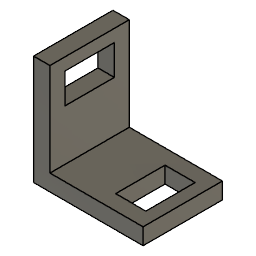
Complete printer assembly (Autodesk Fusion 360 archive; units mm, degrees)
design "T nut L clamp"
part number: 2025-12-24-15-34-34-820
Autodesk Fusion 360 part; units mm, degrees
sketch "Sketch1" plane through (0, 0, 0) normal (0, 1, 0) x (1, 0, 0)
  line L0 (0, 0) -> (3, 0)
  line L1 (3, 0) -> (3, -20)
  line L2 (3, -20) -> (0, -20)
  line L3 (0, -20) -> (0, 0)
  line L4 (0, 0) -> (20, 0)
  line L5 (20, 0) -> (20, -3)
  line L6 (20, -3) -> (0, -3)
  line L7 (0, -3) -> (0, 0)
  dimension "d1" = 20
  dimension "d2" = 3
  dimension "d3" = 20
  dimension "d4" = 3
  constraint horizontal L0
  constraint vertical L1
  constraint horizontal L2
  constraint vertical L3
  constraint coincident L0.start L3.end
  constraint horizontal L4
  constraint vertical L5
  constraint horizontal L6
  constraint vertical L7
  measures "d1" distance of L0 L2
  measures "d2" distance of L4 L6
  measures "d3" distance of L5 L7
  measures "d4" distance of L1 L3
extrude "Extrude1" add sketch "Sketch1" along normal blind 14.5
sketch "Sketch2" plane through (0, 0, 3) normal (0, 0, 1) x (-1, 0, 0)
  line L0 (-3, 0) -> (-20, 0)
  line L1 (-20, 0) -> (-20, -14.5)
  line L2 (-20, -14.5) -> (-3, -14.5)
  line L3 (-3, -14.5) -> (-3, 0)
  line L4 (-12.25, -11.75) -> (-17.75, -11.75)
  line L5 (-17.75, -11.75) -> (-17.75, -2.75)
  line L6 (-17.75, -2.75) -> (-12.25, -2.75)
  line L7 (-12.25, -2.75) -> (-12.25, -11.75)
  dimension "d7" = 5.5
  dimension "d8" = 9
  dimension "d9" = 2.75
  dimension "d10" = 2.25
  constraint horizontal L4
  constraint vertical L5
  constraint horizontal L6
  constraint vertical L7
  measures "d7" distance of L4.start L4.end
  measures "d8" distance of L4 L6
  measures "d9" distance of L0 L6
  measures "d10" distance of L1 L5
extrude "Extrude2" cut sketch "Sketch2" against normal blind 20 contours L4 L5 L6 L7
sketch "Sketch3" plane through (3, 0, 0) normal (1, 0, 0) x (0, 1, 0)
  line L0 (0, 20) -> (0, 3)
  line L1 (0, 3) -> (14.5, 3)
  line L2 (14.5, 3) -> (14.5, 20)
  line L3 (14.5, 20) -> (0, 20)
  line L4 (2.75, 17.75) -> (11.75, 17.75)
  line L5 (11.75, 17.75) -> (11.75, 12.25)
  line L6 (11.75, 12.25) -> (2.75, 12.25)
  line L7 (2.75, 12.25) -> (2.75, 17.75)
  dimension "d13" = 9
  dimension "d14" = 5.5
  dimension "d15" = 2.75
  dimension "d16" = 2.25
  constraint horizontal L4
  constraint vertical L5
  constraint horizontal L6
  constraint vertical L7
  measures "d13" distance of L4.start L4.end
  measures "d14" distance of L4 L6
  measures "d15" distance of L0 L7
  measures "d16" distance of L3 L4
extrude "Extrude3" cut sketch "Sketch3" against normal blind 20 contours L4 L5 L6 L7

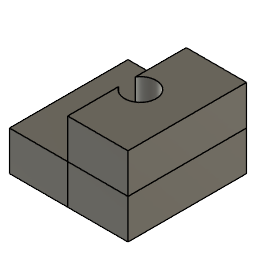
design "Z smooth rod holder"
part number: 2025-12-29-13-48-08-419
Autodesk Fusion 360 part; units mm, degrees
sketch "Sketch1" plane through (0, 0, 0) normal (0, 0, 1) x (1, 0, 0)
  line L0 (0, 0) -> (30, 0)
  line L1 (30, 0) -> (30, 30)
  line L2 (30, 30) -> (0, 30)
  line L3 (0, 30) -> (0, 0)
  circle A0 centre (13, 15) radius 2.75
  circle A1 centre (18.14, 15) radius 4
  line L4 (14.7492, 17.122) -> (14.7492, 12.878)
  line L5 (14.7492, 12.878) -> (14.7492, 0)
  line L6 (14.7492, 0) -> (14.7492, 30)
  dimension "d1" = 30
  dimension "d2" = 30
  dimension "d3" = 5.5
  dimension "d4" = 13
  dimension "d5" = 8
  dimension "d6" = 15
  dimension "d7" = 15
  dimension "d8" = 5.14
  constraint horizontal L0
  constraint vertical L1
  constraint horizontal L2
  constraint vertical L3
  constraint coincident L0.start L3.end
  constraint coincident A1 L4.start
  constraint coincident A0 L4.start
  constraint coincident A1 L4.end
  constraint coincident A0 L4.end
  constraint coincident L0 L5.end
  constraint perpendicular L0 L5
  constraint coincident L2 L6.end
  constraint perpendicular L2 L6
  measures "d1" distance of L1 L3
  measures "d2" distance of L0 L2
  measures "d3" diameter of A0
  measures "d4" distance of L3 A0.centre
  measures "d5" diameter of A1
  measures "d6" distance of L0 A0.centre
  measures "d7" distance of L0 A1.centre
  measures "d8" distance of A0.centre A1.centre
extrude "Extrude1" add sketch "Sketch1" along normal blind 10 contours L0 L2 L3 A0 L5 L6 | L0 L1 L2 A1 L5 L6 makes body 1
extrude "Extrude2" add sketch "Sketch1" along normal blind 20 separate body contours L0 L1 L2 A1 L5 L6 makes body 2

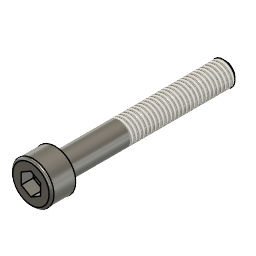
design "Hexagon Socket Head Cap Screw ISO 4762 - M5 x 35 Steel 4.6 Plain"
description: Hexagon Socket Head Cap Screw ISO 4762 - M5 x 35
part number: ISO 4762 - M5 x 35 Steel 4.6 Plain
Autodesk Fusion 360 part; units mm, degrees
sketch "Sketch1" plane through (0, 0, 0) normal (0, 1, 0) x (1, 0, 0)
  line L0 (-2.5, 0) -> (-2.5, 35)
  line L1 (-2.5, 35) -> (0, 35)
  line L2 (0, 35) -> (0, -5)
  line L3 (-2.5, 0) -> (-4.25, 0)
  line L4 (-4.25, 0) -> (-4.25, -5)
  line L5 (-4.25, -5) -> (0, -5)
  dimension "d9" = 5
  dimension "d106" = 5
  dimension "d107" = 35
  dimension "d116" = 8.5
  constraint perpendicular L0 L1
  constraint collinear origin L1.end L2.end
  constraint perpendicular L0 L3
  constraint coincident origin L3
  constraint vertical L2
  constraint coincident L2 L5.end
  constraint perpendicular L2 L5
  measures "d106" distance of L3 L5
  measures "d107" distance of origin L1
revolve "Revolve1" add sketch "Sketch1" angle 360 about axis through (0, 0, -35) along (0, 0, 1)
ref_plane "WorkPlane1" through (0, 0, 5) normal (0, 0, 1) x (1, 0, 0)
sketch "Sketch6" plane through (0, 0, 5) normal (0, 0, 1) x (1, 0, 0)
  line L0 (-2, 1.1547) -> (-2, -1.1547)
  line L1 (-2, -1.1547) -> (0, -2.3094)
  line L2 (0, -2.3094) -> (2, -1.1547)
  line L3 (2, -1.1547) -> (2, 1.1547)
  line L4 (2, 1.1547) -> (0, 2.3094)
  line L5 (0, 2.3094) -> (-2, 1.1547)
  dimension "d117" = 4
  constraint vertical L0
  measures "d117" distance of L0 L3
extrude "Extrude1" cut sketch "Sketch6" against normal blind 2.5
extrude "Extrude2" cut 1 faces at (0.6667, -0.3849, 2.5) along direction (0, 0, -1) blind 2.5 draft -85
fillet "Fillet4" radius 0.5 1 edges at (-3.9624, 1.5369, 5)
thread "Thread3" "ISO Metric profile 5.0 M5x0.8 M5x0.8 6g" major diameter 4.901 minor diameter 3.9895 pitch 0.8 angle 60 resizes the face on face at (-2.4969, 0.1246, -23.3333) from (0, 0, -13) to (0, 0, -35)
sketch "Sketch7" plane through (0, 0, 0) normal (0, 1, 0) x (1, 0, 0)
  line L0 (-2.55, 35) -> (-2.55, 34.5)
  line L1 (-2.55, 34.5) -> (-2.05, 35)
  line L2 (0, 35) -> (0, -5)
  line L3 (-2.55, 35) -> (0, 35)
  dimension "d101" = 45
  dimension "d112" = 0.5
  dimension "d113" = 2.55
  constraint coincident L2.start L3.end
  constraint perpendicular L2 L3
  constraint coincident L1.end L3
  constraint perpendicular L0 L3
  measures "d101" angle of L0 L1
  measures "d112" distance of L0.end L3
  measures "d113" distance of L0 L2.start
revolve "Revolve3" cut sketch "Sketch7" angle 360 about axis through (0, 0, 1.75) along (0, 0, 1)
equation "d9 = adsk_nomdia"
equation "adsk_nomlen = 35.00 mm"
equation "adsk_headh = 5.00 mm"
equation "adsk_headdia = 8.50 mm"
equation "adsk_nomdia = 5.00 mm"
equation "adsk_philwidth = 4.00 mm"
equation "d31 = -adsk_phildepth"
equation "adsk_phildepth = 2.50 mm"
equation "d71 = adsk_headh"
equation "d76 = -adsk_phildepth"
equation "adsk_thrlen = 22.00 mm"
equation "d86 = adsk_nomdia * 0.1"
equation "adsk_startang = 45.00 deg"
equation "d101 = adsk_startang"
equation "adsk_pitch1 = 0.80 mm"
equation "adsk_startlen = 0.50 mm"
equation "d106 = adsk_headh"
equation "d107 = adsk_nomlen"
equation "d112 = adsk_startlen"
equation "d113 = adsk_nomdia * 0.51"
equation "d115 = min(adsk_thrlen; adsk_nomlen - 0.001 mm)"
equation "d116 = adsk_headdia"
equation "d117 = adsk_philwidth"

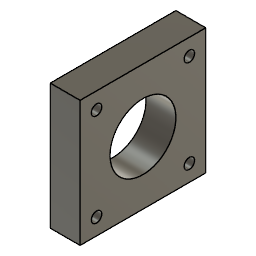
design "Nema 17 face mount"
part number: 2025-12-27-18-46-16-654
Autodesk Fusion 360 part; units mm, degrees
sketch "Sketch1" plane through (0, 0, 0) normal (1, 0, 0) x (0, 1, 0)
  line L0 (5, 30) -> (25, 30)
  line L1 (25, 30) -> (25, 0)
  line L2 (25, 0) -> (5, 0)
  line L3 (5, 0) -> (5, 30)
  circle A0 centre (15, 15) radius 4
  dimension "d1" = 8
  dimension "d2" = 10
  dimension "d3" = 20
  dimension "d4" = 15
  dimension "d5" = 15
  dimension "d6" = 30
  constraint horizontal L0
  constraint vertical L1
  constraint horizontal L2
  constraint vertical L3
  measures "d1" diameter of A0
  measures "d2" distance of L1 A0.centre
  measures "d3" distance of L1 L3
  measures "d4" distance of L2 A0.centre
  measures "d5" distance of L0 A0.centre
  measures "d6" distance of L0 L2
sketch "Sketch2" plane through (0, 0, 0) normal (1, 0, 0) x (0, 1, 0)
  line L0 (0, 0) -> (42, 0)
  line L1 (42, 0) -> (42, 42)
  line L2 (42, 42) -> (0, 42)
  line L3 (0, 42) -> (0, 0)
  circle A0 centre (21, 21) radius 11
  circle A1 centre (5.5, 36.5) radius 1.75
  circle A2 centre (36.5, 36.5) radius 1.75
  circle A3 centre (5.5, 5.5) radius 1.75
  circle A4 centre (36.5, 5.5) radius 1.75
  dimension "d9" = 42
  dimension "d10" = 42
  dimension "d11" = 22
  dimension "d12" = 3.5
  dimension "d13" = 3.5
  dimension "d14" = 3.5
  dimension "d15" = 3.5
  dimension "d16" = 5.5
  dimension "d17" = 5.5
  dimension "d18" = 5.5
  dimension "d19" = 5.5
  dimension "d20" = 5.5
  dimension "d21" = 5.5
  dimension "d22" = 5.5
  dimension "d23" = 5.5
  dimension "d24" = 21
  dimension "d25" = 21
  constraint horizontal L0
  constraint vertical L1
  constraint horizontal L2
  constraint vertical L3
  constraint coincident L0.start L3.end
  measures "d9" distance of L0.start L2.end
  measures "d10" distance of L1 L3
  measures "d11" diameter of A0
  measures "d12" diameter of A1
  measures "d13" diameter of A2
  measures "d14" diameter of A3
  measures "d15" diameter of A4
  measures "d16" distance of L1 A2.centre
  measures "d17" distance of L2 A2.centre
  measures "d18" distance of L2 A1.centre
  measures "d19" distance of L3 A1.centre
  measures "d20" distance of L3 A3.centre
  measures "d21" distance of L0 A3.centre
  measures "d22" distance of L0 A4.centre
  measures "d23" distance of L1 A4.centre
  measures "d24" distance of L3 A0.centre
  measures "d25" distance of L0 A0.centre
extrude "Extrude2" add sketch "Sketch2" along normal blind 10

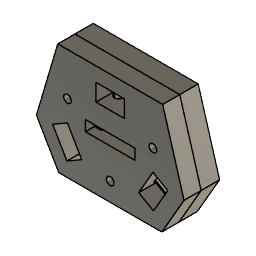
design "#d printer extruder coupling"
part number: 2025-12-16-20-43-48-911
Autodesk Fusion 360 part; units mm, degrees
sketch "Sketch1" plane through (0, 0, 0) normal (0, 1, 0) x (1, 0, 0)
  line L0 (36.1658, 0) -> (0, 0)
  line L1 (0, 0) -> (-15.6882, -27.1727)
  line L2 (-15.6882, -27.1727) -> (-0.6882, -78)
  line L3 (-0.6882, -78) -> (36.1658, -78)
  line L4 (36.1658, -78) -> (36.1658, 0)
  line L5 (36.1658, -68) -> (26.1658, -68)
  line L6 (26.1658, -68) -> (26.1658, -56)
  line L7 (26.1658, -56) -> (36.1658, -56)
  line L8 (36.1658, -56) -> (36.1658, -68)
  line L9 (6.1658, -33.3205) -> (16.1658, -16)
  line L10 (16.1658, -16) -> (5.7735, -10)
  line L11 (5.7735, -10) -> (-4.2265, -27.3205)
  line L12 (-4.2265, -27.3205) -> (6.1658, -33.3205)
  line L13 (72.3316, 0) -> (88.0198, -27.1727)
  line L14 (36.1658, -56) -> (36.1658, -68)
  line L15 (73.0198, -78) -> (36.1658, -78)
  line L16 (36.1658, -68) -> (46.1658, -68)
  line L17 (36.1658, 0) -> (72.3316, 0)
  line L18 (76.5581, -27.3205) -> (66.1658, -33.3205)
  line L19 (88.0198, -27.1727) -> (73.0198, -78)
  line L20 (46.1658, -56) -> (36.1658, -56)
  line L21 (46.1658, -68) -> (46.1658, -56)
  line L22 (66.1658, -33.3205) -> (56.1658, -16)
  line L23 (36.1658, -78) -> (36.1658, 0)
  line L24 (66.5581, -10) -> (76.5581, -27.3205)
  line L25 (56.1658, -16) -> (66.5581, -10)
  point P0 (72.3316, 0)
  dimension "d1" = 10
  dimension "d2" = 12
  dimension "d5" = 12
  dimension "d6" = 20
  dimension "d7" = 10
  dimension "d8" = 10
  dimension "d9" = 40
  dimension "d10" = 10
  dimension "d11" = 26.854
  dimension "d12" = 15
  dimension "d13" = 36.1658
  dimension "d14" = 10
  dimension "d15" = 78
  dimension "d16" = 73.708
  dimension "d17" = 72.3316
  constraint coincident L0.end L1.start
  constraint horizontal L0
  constraint parallel L0 L3
  constraint perpendicular L0 L4
  constraint horizontal L5
  constraint vertical L6
  constraint horizontal L7
  constraint vertical L8
  constraint coincident L4 L5.start
  constraint parallel L1 L11
  constraint parallel L9 L11
  constraint perpendicular L9 L12
  constraint symmetric L0.end L4 L13.start
  constraint symmetric L0.start L4 L17.start
  constraint symmetric L0.end L4 P0
  constraint symmetric L1.end L4 L13.end
  constraint symmetric L2.end L4 L15.start
  constraint symmetric L3.end L4 L15.end
  constraint symmetric L4 L5.start L8.end
  constraint symmetric L4 L5.end L16.end
  constraint symmetric L4 L6.end L20.start
  constraint symmetric L4 L7.end L8.start
  constraint symmetric L4 L9.start L18.end
  constraint symmetric L4 L9.end L22.end
  constraint symmetric L4 L10.end L24.start
  constraint symmetric L4 L11.end L18.start
  measures "d1" distance of L5.start L5.end
  measures "d2" distance of L5 L7
  measures "d5" distance of L9.start L11.end
  measures "d6" distance of L10 L12
  measures "d7" distance of L1 L11
  measures "d8" distance of L0 L10.end
  measures "d9" distance of L7 L9.end
  measures "d10" distance of L6 L9.end
  measures "d11" distance of L2.end L6
  measures "d12" horizontal distance of L1.end L2.end
  measures "d13" distance of L0.end L0.start
  measures "d14" distance of L3 L5
  measures "d15" distance of L0 L3
  measures "d16" distance of L2.end L15.start
  measures "d17" distance of L0.end L13.start
extrude "Extrude1" add sketch "Sketch1" along normal blind 25 contours L0 L1 L2 L3 L4 L5 L6 L7 L23 | L4 L13 L15 L16 L17 L19 L20 L21 L23 | L4 L8 L14 L16 L20 L21 L23 | L4 L5 L6 L7 L8 L14 L23 | L9 L10 L11 L12 | L18 L22 L24 L25 makes body 1
extrude "Extrude2" cut sketch "Sketch1" along normal blind 15 contours L4 L8 L14 L16 L20 L21 L23 | L4 L5 L6 L7 L8 L14 L23 | L9 L10 L11 L12 | L18 L22 L24 L25 bodies 1
sketch "Sketch2" plane through (0, 0, 78) normal (0, 0, 1) x (-1, 0, 0)
  line L0 (0.6882, 0) -> (-73.0198, 0)
  line L1 (-73.0198, 0) -> (-73.0198, -25)
  line L2 (-73.0198, -25) -> (0.6882, -25)
  line L3 (0.6882, -25) -> (0.6882, 0)
  line L4 (-26.1658, -9) -> (-46.1658, -9)
  line L5 (-46.1658, -9) -> (-46.1658, -15)
  line L6 (-46.1658, -15) -> (-26.1658, -15)
  line L7 (-26.1658, -15) -> (-26.1658, -9)
  circle A0 centre (-30.1658, -12) radius 3
  circle A1 centre (-42.1658, -12) radius 3
  line L8 (0.6882, 0) -> (-36.1658, 0)
  dimension "d22" = 20
  dimension "d23" = 6
  dimension "d24" = 6
  dimension "d25" = 6
  dimension "d26" = 12
  dimension "d27" = 3
  dimension "d28" = 3
  dimension "d29" = 4
  dimension "d30" = 9
  dimension "d31" = 26.854
  constraint horizontal L4
  constraint vertical L5
  constraint horizontal L6
  constraint vertical L7
  measures "d22" distance of L4.start L4.end
  measures "d23" distance of L4 L6
  measures "d24" diameter of A0
  measures "d25" diameter of A1
  measures "d26" distance of A0.centre A1.centre
  measures "d27" distance of L6 A0.centre
  measures "d28" distance of L4 A1.centre
  measures "d29" distance of L7 A0.centre
  measures "d30" distance of L4 L8
  measures "d31" distance of L3 L7
extrude "Extrude3" add sketch "Sketch2" against normal blind 30 contours L4 L6 L7 A0 | L4 L6 A0 A1 | L4 L5 L6 A1 bodies 1
sketch "Sketch3" plane through (0, 0, 0) normal (-0.866025, 0, -0.5) x (0, -1, 0)
  line L0 (0, 0) -> (0, 31.3764)
  line L1 (0, 31.3764) -> (-25, 31.3764)
  line L2 (-25, 31.3764) -> (-25, 0)
  line L3 (-25, 0) -> (0, 0)
  line L4 (-15, 25.7735) -> (-9, 25.7735)
  line L5 (-9, 25.7735) -> (-9, 5.7735)
  line L6 (-9, 5.7735) -> (-15, 5.7735)
  line L7 (-15, 5.7735) -> (-15, 25.7735)
  circle A0 centre (-12, 21.7735) radius 3
  circle A1 centre (-12, 9.7735) radius 3
  line L8 (0, 0) -> (0, 31.3764)
  point P0 (0, 5.7735)
  dimension "d34" = 6
  dimension "d35" = 20
  dimension "d36" = 6
  dimension "d37" = 6
  dimension "d38" = 12
  dimension "d39" = 4
  dimension "d40" = 3
  dimension "d41" = 9
  dimension "d42" = 5.7735
  dimension "d43" = 5.7735
  dimension "d44" = 3
  constraint horizontal L4
  constraint vertical L5
  constraint horizontal L6
  constraint vertical L7
  measures "d34" distance of L4.start L4.end
  measures "d35" distance of L4 L6
  measures "d36" diameter of A0
  measures "d37" diameter of A1
  measures "d38" distance of A0.centre A1.centre
  measures "d39" distance of L4 A0.centre
  measures "d40" distance of L7 A1.centre
  measures "d41" distance of L5 L8
  measures "d42" distance of L3 P0
  measures "d43" distance of L3 L6
  measures "d44" distance of L5 A0.centre
extrude "Extrude4" add sketch "Sketch3" against normal blind 30 contours L4 L5 L7 A0 | L5 L7 A0 A1 | L5 L6 L7 A1 bodies 1
sketch "Sketch4" plane through (54.2487, 0, -31.3205) normal (0.866025, 0, -0.5) x (0, 1, 0)
  line L0 (0, 67.5422) -> (0, 36.1658)
  line L1 (0, 36.1658) -> (25, 36.1658)
  line L2 (25, 36.1658) -> (25, 67.5422)
  line L3 (25, 67.5422) -> (0, 67.5422)
  line L4 (15, 61.9393) -> (9, 61.9393)
  line L5 (9, 61.9393) -> (9, 41.9393)
  line L6 (9, 41.9393) -> (15, 41.9393)
  line L7 (15, 41.9393) -> (15, 61.9393)
  circle A0 centre (12, 57.9393) radius 3
  circle A1 centre (12, 45.9393) radius 3
  line L8 (0, 36.1658) -> (0, 67.5422)
  point P0 (0, 61.9393)
  point P1 (0, 67.5422)
  dimension "d47" = 5.6029
  dimension "d50" = 6
  dimension "d51" = 20
  dimension "d52" = 6
  dimension "d53" = 6
  dimension "d54" = 3
  dimension "d55" = 3
  dimension "d56" = 4
  dimension "d57" = 4
  dimension "d58" = 12
  dimension "d59" = 9
  dimension "d60" = 0
  constraint horizontal L4
  constraint vertical L5
  constraint horizontal L6
  constraint vertical L7
  measures "d47" distance of P0 P1
  measures "d50" distance of L4.start L4.end
  measures "d51" distance of L4 L6
  measures "d52" diameter of A0
  measures "d53" diameter of A1
  measures "d54" distance of L5 A0.centre
  measures "d55" distance of L5 A1.centre
  measures "d56" distance of L4 A0.centre
  measures "d57" distance of L6 A1.centre
  measures "d58" distance of A0.centre A1.centre
  measures "d59" distance of L5 L8
  measures "d60" distance of P0 L4
extrude "Extrude5" add sketch "Sketch4" against normal blind 30 contours L4 L5 L7 A0 | L5 L7 A0 A1 | L5 L6 L7 A1 bodies 1
sketch "Sketch5" plane through (0, 0, 78) normal (0, 0, 1) x (-1, 0, 0)
  line L0 (-30.165, -12) -> (33.5874, -12)
  line L1 (-30.165, -12) -> (-111.0863, -12)
  constraint horizontal L0
  constraint parallel L0 L1
sketch "Sketch6" plane through (0, 0, 0) normal (0, 1, 0) x (1, 0, 0)
  line L0 (73.0198, -78) -> (36.1658, -78)
  line L1 (36.1658, -68) -> (46.1658, -68)
  dimension "d63" = 10
  measures "d63" distance of L0 L1
extrude "Extrude6" cut sketch "Sketch2" against normal blind 16 from surface at -8 contours A0 | A1 bodies 1
extrude "Extrude7" cut sketch "Sketch3" against normal blind 16 from surface at -8 contours A0 | A1 bodies 1
extrude "Extrude8" cut sketch "Sketch4" against normal blind 16 from surface at -8 contours A0 | A1 bodies 1
sketch "Sketch7" plane through (0, 0, 0) normal (0, 1, 0) x (1, 0, 0)
  circle A0 centre (6.1658, -48) radius 2.7
  circle A1 centre (66.1658, -48) radius 2.7
  circle A2 centre (36.1658, -13) radius 2.7
  line L0 (36.1658, -78) -> (36.1658, 0)
  line L1 (36.1658, -68) -> (46.1658, -68)
  line L2 (-15.6882, -27.1727) -> (-0.6882, -78)
  line L3 (88.0198, -27.1727) -> (73.0198, -78)
  line L4 (36.1658, 0) -> (72.3316, 0)
  point P0 (26.1658, -68)
  dimension "d73" = 5.4
  dimension "d74" = 5.4
  dimension "d75" = 5.4
  dimension "d76" = 30
  dimension "d77" = 20
  dimension "d78" = 20
  dimension "d79" = 30
  dimension "d80" = 15.0652
  dimension "d81" = 15.0652
  dimension "d82" = 13
  constraint coincident A2.centre L0
  measures "d73" diameter of A0
  measures "d74" diameter of A1
  measures "d75" diameter of A2
  measures "d76" distance of A0.centre L0
  measures "d77" vertical distance of A0.centre P0
  measures "d78" distance of A1.centre L1
  measures "d79" distance of A1.centre L0
  measures "d80" distance of A0.centre L2
  measures "d81" distance of A1.centre L3
  measures "d82" distance of A2.centre L4
extrude "Extrude9" cut sketch "Sketch7" along normal blind 80 bodies 1
extrude "Extrude10" cut sketch "Sketch1" along normal blind 12 contours L4 L8 L14 L16 L20 L21 L23 | L4 L5 L6 L7 L8 L14 L23 | L9 L10 L11 L12 | L18 L22 L24 L25 bodies 1
split "Split1" by curves path "Sketch5" along L1 L0 bodies 1 makes body 2 at (36.2331, 25, 36.9625)
move_body "Move1" bodies 1 to x (1, 0, 0) y (0, 1, 0) z (0, 0, 1) at (0, -40, 0)
move_body "Move2" bodies 1 to x (1, 0, 0) y (0, 1, 0) z (0, 0, 1) at (0, 40, 0)
extrude "Extrude11" cut sketch "Sketch4" against normal blind 20 from surface at -6 contours A0 | A1 bodies 1 2
extrude "Extrude12" cut sketch "Sketch3" against normal blind 20 from surface at -6 contours A0 | A1 bodies 1 2
extrude "Extrude13" cut sketch "Sketch2" against normal blind 20 from surface at -6 contours A0 | A1 bodies 1 2
sketch "Sketch9" plane through (0, 0, 0) normal (0, -1, 0) x (1, 0, 0)
  circle A0 centre (36.1658, 13) radius 2.7
  circle A1 centre (6.1658, 48) radius 2.7
  circle A2 centre (66.1658, 48) radius 2.7
  line L0 (5.7735, 10) -> (-4.2265, 27.3205)
  line L1 (-4.2265, 27.3205) -> (6.1658, 33.3205)
  line L2 (6.1658, 33.3205) -> (16.1658, 16)
  line L3 (16.1658, 16) -> (5.7735, 10)
  line L4 (26.1658, 56) -> (26.1658, 68)
  line L5 (26.1658, 68) -> (46.1658, 68)
  line L6 (46.1658, 68) -> (46.1658, 56)
  line L7 (46.1658, 56) -> (26.1658, 56)
  line L8 (66.5581, 10) -> (56.1658, 16)
  line L9 (56.1658, 16) -> (66.1658, 33.3205)
  line L10 (66.1658, 33.3205) -> (76.5581, 27.3205)
  line L11 (76.5581, 27.3205) -> (66.5581, 10)
  line L12 (0, 0) -> (72.3316, 0)
  line L13 (72.3316, 0) -> (88.0198, 27.1727)
  line L14 (88.0198, 27.1727) -> (73.0198, 78)
  line L15 (73.0198, 78) -> (-0.6882, 78)
  line L16 (-0.6882, 78) -> (-15.6882, 27.1727)
  line L17 (-15.6882, 27.1727) -> (0, 0)
  line L18 (18.7658, 41.7) -> (53.5658, 41.7)
  line L19 (53.5658, 41.7) -> (53.5658, 34.3)
  line L20 (53.5658, 34.3) -> (18.7658, 34.3)
  line L21 (18.7658, 34.3) -> (18.7658, 41.7)
  circle A3 centre (21.2658, 38) radius 1.25
  circle A4 centre (51.0658, 38) radius 1.25
  line L22 (23.7658, 41.7) -> (48.5658, 41.7)
  line L23 (48.5658, 41.7) -> (48.5658, 34.3)
  line L24 (48.5658, 34.3) -> (23.7658, 34.3)
  line L25 (23.7658, 34.3) -> (23.7658, 41.7)
  point P0 (6.1658, 48)
  point P1 (66.1658, 48)
  dimension "d96" = 7.4
  dimension "d97" = 34.8
  dimension "d98" = 2.5
  dimension "d99" = 2.5
  dimension "d100" = 15.1
  dimension "d101" = 15.1
  dimension "d102" = 29.8
  dimension "d103" = 7.4
  dimension "d104" = 7.4
  dimension "d105" = 24.8
  dimension "d106" = 3.7
  dimension "d107" = 3.7
  dimension "d108" = 10
  dimension "d109" = 2.5
  dimension "d110" = 5
  dimension "d111" = 5
  constraint horizontal L18
  constraint vertical L19
  constraint horizontal L20
  constraint vertical L21
  constraint horizontal L22
  constraint vertical L23
  constraint horizontal L24
  constraint vertical L25
  constraint coincident L20 L23.end
  measures "d96" distance of L18 L20
  measures "d97" distance of L19 L21
  measures "d98" diameter of A3
  measures "d99" diameter of A4
  measures "d100" horizontal distance of A3.centre P0
  measures "d101" horizontal distance of A4.centre P1
  measures "d102" horizontal distance of A3.centre A4.centre
  measures "d103" distance of L20 L22
  measures "d104" distance of L22 L24
  measures "d105" distance of L23 L25
  measures "d106" distance of L20 A3.centre
  measures "d107" distance of L20 A4.centre
  measures "d108" vertical distance of A3.centre P0
  measures "d109" distance of L21 A3.centre
  measures "d110" distance of L21 L25
  measures "d111" distance of L19 L23
extrude "Extrude14" cut sketch "Sketch9" against normal blind 2.5 contours L18 L20 L21 L25 | L18 L20 L22 L23 L24 L25 | L18 L19 L20 L23 | A3 | A4 bodies 1
extrude "Extrude15" cut sketch "Sketch9" against normal blind 6.4 contours L18 L20 L22 L23 L24 L25 bodies 1
extrude "Extrude16" cut sketch "Sketch9" against normal blind 30 contours A3 | A4 bodies 1 2
extrude "Extrude17" cut sketch "Sketch9" against normal blind 26 contours L18 L20 L22 L23 L24 L25 bodies 1 2
extrude "Extrude18" cut sketch "Sketch9" against normal blind 6.4 contours L18 L20 L21 L25 | L18 L19 L20 L23 bodies 1
move_body "Move3" bodies 1 to x (1, 0, 0) y (0, 0, 1) z (0, -1, 0) at (0, -35, 0)
move_body "Move4" bodies 2 to x (1, 0, 0) y (0, 0, -1) z (0, 1, 0) at (0, 2, 12)
move_body "Move5" bodies 1 to x (1, 0, 0) y (0, 0, -1) z (0, 1, 0) at (0, -113, -38)
move_body "Move6" bodies 2 to x (1, 0, 0) y (0, 0, 1) z (0, -1, 0) at (0, -96, -5)
move_body "Move7" bodies 2 to x (1, 0, 0) y (0, 1, 0) z (0, 0, 1) at (0, -5, 0)
equation "d43 = d42"

design "Hexagon Regular Nut DIN EN ISO 4032 - M5 Steel 6 Plain"
description: Hexagon Regular Nut DIN EN ISO 4032 - M5
part number: DIN EN ISO 4032 - M5 Steel 6 Plain
Autodesk Fusion 360 part; units mm, degrees
sketch "Sketch1" plane through (0, 0, 0) normal (0, 1, 0) x (1, 0, 0)
  line L0 (0, 0) -> (0, -4.7)
  line L1 (-2.5, 0) -> (-3.92, 0)
  line L2 (-3.92, 0) -> (-4.62, -0.4041)
  line L3 (-4.62, -0.4041) -> (-4.62, -4.2959)
  line L4 (-4.62, -4.2959) -> (-3.92, -4.7)
  line L5 (-3.92, -4.7) -> (-2.5, -4.7)
  line L6 (-2.5, -4.7) -> (-2.5, 0)
  dimension "d121" = 5
  dimension "d122" = 30
  dimension "d123" = 30
  dimension "d128" = 9.24
  dimension "d172" = 7.84
  dimension "d179" = 4.7
  constraint vertical L0
  constraint coincident L0 L0.end
  constraint coincident origin L0
  constraint horizontal L1
  constraint coincident L0.start L1
  constraint coincident L0.start origin
  constraint coincident L0.end L5
  constraint vertical L1.end L4.end
  measures "d122" angle of L1 L2
  measures "d123" angle of L4 L5
  measures "d179" distance of L1 L5
revolve "Revolve1" add sketch "Sketch1" angle 360 about axis through (0, 0, 0) along (0, 0, 1)
sketch "Sketch8" plane through (0, 0, 4.7) normal (0, 0, 1) x (1, 0, 0)
  line L0 (-4, -2.3118) -> (-4, 2.3118)
  circle A0 centre (0, 0) radius 2.5
  circle A1 centre (0, 0) radius 4.62
  dimension "d114" = 4
  constraint coincident L0.end A1
  constraint coincident L0.start A1
  constraint vertical L0
  measures "d114" distance of A0.centre L0
extrude "Extrude5" cut sketch "Sketch8" against normal blind 4.7 contours L0 A1 picked at (-4.1, -0.5631)
pattern_circular "C-Pattern2" count 6 over 360 about axis through (0, 0, 1.75) along (0, 0, 1) of "Extrude5"
thread "Thread3" "ISO Metric profile 5.0 M5x0.8 M5x0.8 6H" major diameter 5.12 minor diameter 4.234 pitch 0.8 angle 60 resizes the face on face at (-2.4876, 0.2489, 3.1333)
sketch "Sketch12" plane through (0, 0, 0) normal (0, 1, 0) x (1, 0, 0)
  line L0 (-2.5, 0) -> (0, 0)
  line L1 (-1.1432, -2.35) -> (-2.5, 0)
  line L2 (-2.5, -4.7) -> (0, -4.7)
  line L3 (-1.1432, -2.35) -> (-2.5, -4.7)
  line L4 (0, 0) -> (0, -4.7)
  dimension "d169" = 60
  dimension "d177" = 2.5
  dimension "d178" = 60
  constraint horizontal L0
  constraint coincident L1.start L3.start
  constraint vertical L0.start L2.start
  constraint coincident L2.end L4.end
  constraint coincident L0.end L4.start
  constraint perpendicular L2 L4
  measures "d169" angle of L2 L3
  measures "d177" distance of L0.start L4
  measures "d178" angle of L0 L1
revolve "Revolve3" cut sketch "Sketch12" angle 360 about axis through (0, 0, 1.75) along (0, 0, 1)
equation "adsk_nheig = 4.70 mm"
equation "adsk_maxdia = 9.24 mm"
equation "adsk_nomdia = 5.00 mm"
equation "d89 = -adsk_nheig"
equation "adsk_waflat = 8.00 mm"
equation "d114 = adsk_waflat / 2"
equation "adsk_chamang1 = 30.00 deg"
equation "adsk_chamang2 = 30.00 deg"
equation "d121 = adsk_nomdia"
equation "d122 = adsk_chamang1"
equation "d123 = adsk_chamang2"
equation "d128 = adsk_maxdia"
equation "d163 = adsk_nheig"
equation "adsk_beardia = 7.84 mm"
equation "d172 = adsk_beardia"
equation "d177 = adsk_nomdia * 0.5"
equation "d179 = adsk_nheig"

design "Y carriage idler pulley"
part number: 2025-12-10-15-46-54-100
Autodesk Fusion 360 part; units mm, degrees
other "DerivedContext1"
other "DerivedContext2"
sketch "Sketch7" plane through (0, 0, 0) normal (0, 0, 1) x (1, 0, 0)
  line L0 (0, 0) -> (93, 0)
  line L1 (93, 0) -> (93, 78)
  line L2 (93, 78) -> (0, 78)
  line L3 (0, 78) -> (0, 0)
  circle A0 centre (15, 30) radius 2.1
  circle A1 centre (15, 48) radius 2.1
  circle A2 centre (39, 48) radius 2.1
  circle A3 centre (39, 30) radius 2.1
  circle A4 centre (54, 48) radius 2.1
  circle A5 centre (78, 48) radius 2.1
  circle A6 centre (54, 30) radius 2.1
  circle A7 centre (78, 30) radius 2.1
  line L4 (17, 20) -> (37, 20)
  line L5 (37, 20) -> (37, 10)
  line L6 (37, 10) -> (17, 10)
  line L7 (17, 10) -> (17, 20)
  line L8 (56, 68) -> (76, 68)
  line L9 (76, 68) -> (76, 58)
  line L10 (76, 58) -> (56, 58)
  line L11 (56, 58) -> (56, 68)
  line L12 (55, 0) -> (85, 0)
  line L13 (86, 0) -> (44, 0)
  line L14 (44, 20) -> (86, 20)
  line L15 (86, 20) -> (86, 10)
  line L16 (86, 10) -> (44, 10)
  line L17 (44, 10) -> (44, 20)
  dimension "d16" = 4.2
  dimension "d17" = 4.2
  dimension "d18" = 4.2
  dimension "d19" = 4.2
  dimension "d20" = 4.2
  dimension "d22" = 4.2
  dimension "d23" = 4.2
  dimension "d24" = 4.2
  dimension "d25" = 18
  dimension "d26" = 18
  dimension "d27" = 18
  dimension "d28" = 18
  dimension "d29" = 24
  dimension "d30" = 24
  dimension "d31" = 24
  dimension "d32" = 24
  dimension "d38" = 15
  dimension "d39" = 15
  dimension "d40" = 15
  dimension "d41" = 15
  dimension "d43" = 15
  dimension "d44" = 15
  dimension "d68" = 93
  dimension "d69" = 20
  dimension "d70" = 20
  dimension "d71" = 10
  dimension "d72" = 10
  dimension "d74" = 17
  dimension "d76" = 10
  dimension "d80" = 10
  dimension "d82" = 10
  dimension "d89" = 30
  dimension "d90" = 30
  dimension "d94" = 30
  dimension "d95" = 30
  dimension "d97" = 78
  dimension "d103" = 58
  dimension "d104" = 78
  dimension "d119" = 30
  dimension "d131" = 42
  dimension "d132" = 10
  dimension "d133" = 7
  dimension "d134" = 10
  dimension "d135" = 10
  dimension "d136" = 30
  dimension "d143" = 17
  constraint horizontal L0
  constraint vertical L1
  constraint horizontal L2
  constraint vertical L3
  constraint coincident L0.start L3.end
  constraint horizontal L4
  constraint vertical L5
  constraint horizontal L6
  constraint vertical L7
  constraint horizontal L8
  constraint vertical L9
  constraint horizontal L10
  constraint vertical L11
  constraint horizontal L12
  constraint coincident L0 L12.start
  constraint horizontal L13
  constraint coincident L0 L13.start
  constraint horizontal L14
  constraint vertical L15
  constraint horizontal L16
  constraint vertical L17
  measures "d16" diameter of A0
  measures "d17" diameter of A1
  measures "d18" diameter of A2
  measures "d19" diameter of A3
  measures "d20" diameter of A4
  measures "d22" diameter of A5
  measures "d23" diameter of A6
  measures "d24" diameter of A7
  measures "d25" vertical distance of A0.centre A1.centre
  measures "d26" vertical distance of A2.centre A3.centre
  measures "d27" vertical distance of A4.centre A6.centre
  measures "d28" vertical distance of A5.centre A7.centre
  measures "d29" distance of A0.centre A3.centre
  measures "d30" distance of A1.centre A2.centre
  measures "d31" horizontal distance of A6.centre A7.centre
  measures "d32" horizontal distance of A4.centre A5.centre
  measures "d38" distance of L3 A0.centre
  measures "d39" distance of L3 A1.centre
  measures "d40" distance of A3.centre A6.centre
  measures "d41" distance of A2.centre A4.centre
  measures "d43" distance of L1 A7.centre
  measures "d44" distance of L1 A5.centre
  measures "d68" distance of L1 L3
  measures "d69" distance of L9 L11
  measures "d70" distance of L5 L7
  measures "d71" distance of L4 L6
  measures "d72" distance of L8 L10
  measures "d74" distance of L3 L7
  measures "d76" distance of A0.centre L4
  measures "d80" distance of A5.centre L10
  measures "d82" distance of L2 L8
  measures "d89" distance of L2 A2.centre
  measures "d90" distance of L2 A4.centre
  measures "d94" distance of L2 A1.centre
  measures "d95" distance of L2 A5.centre
  measures "d97" distance of L0 L2
  measures "d103" distance of L2 L4
  measures "d104" distance of L0 L2
  measures "d119" distance of A7.centre L12
  measures "d131" distance of L14.start L14.end
  measures "d132" distance of L14 L16
  measures "d133" distance of L5 L17
  measures "d134" distance of A6.centre L14
  measures "d135" distance of L13 L16
  measures "d136" distance of L0 A0.centre
  measures "d143" distance of L1 L9
extrude "Extrude4" add sketch "Sketch7" along normal blind 8 contours L0 L1 L2 L3 L12 L13 | L4 L5 L6 L7 | L8 L9 L10 L11 | L14 L15 L16 L17
extrude "Extrude6" add sketch "Sketch7" along normal blind 48 from surface at 5 contours L4 L5 L6 L7 | L8 L9 L10 L11
extrude "Extrude7" add sketch "Sketch7" along normal blind 48 from surface at 5 contours L14 L15 L16 L17
sketch "Sketch9" plane through (0, 0, 0) normal (0, 1, 0) x (1, 0, 0)
  circle A0 centre (65, -32) radius 11.05
  circle A1 centre (49.5, -47.5) radius 1.75
  circle A2 centre (80.5, -47.5) radius 1.75
  circle A3 centre (49.5, -16.5) radius 1.75
  circle A4 centre (80.5, -16.5) radius 1.75
  line L0 (44, -8) -> (44, -53)
  line L1 (86, -8) -> (86, -53)
  line L2 (44, -53) -> (86, -53)
  line L3 (0, -8) -> (93, -8)
  dimension "d150" = 22.1
  dimension "d151" = 3.5
  dimension "d152" = 3.5
  dimension "d153" = 3.5
  dimension "d154" = 3.5
  dimension "d155" = 21
  dimension "d156" = 21
  dimension "d157" = 21
  dimension "d158" = 24
  dimension "d159" = 31
  dimension "d160" = 31
  dimension "d161" = 31
  dimension "d162" = 31
  dimension "d163" = 15.5
  dimension "d164" = 15.5
  dimension "d165" = 15.5
  dimension "d166" = 15.5
  dimension "d167" = 15.5
  measures "d150" diameter of A0
  measures "d151" diameter of A1
  measures "d152" diameter of A2
  measures "d153" diameter of A3
  measures "d154" diameter of A4
  measures "d155" distance of A0.centre L0
  measures "d156" distance of A0.centre L1
  measures "d157" distance of A0.centre L2
  measures "d158" distance of A0.centre L3
  measures "d159" horizontal distance of A1.centre A2.centre
  measures "d160" horizontal distance of A3.centre A4.centre
  measures "d161" vertical distance of A2.centre A4.centre
  measures "d162" vertical distance of A1.centre A3.centre
  measures "d163" horizontal distance of A0.centre A1.centre
  measures "d164" horizontal distance of A0.centre A2.centre
  measures "d165" horizontal distance of A0.centre A4.centre
  measures "d166" vertical distance of A0.centre A3.centre
  measures "d167" vertical distance of A0.centre A2.centre
extrude "Extrude8" cut sketch "Sketch9" along normal blind 30 contours A0 | A1 | A2 | A3 | A4
extrude "Extrude9" add sketch "Sketch7" along normal blind 63 from surface at 5 contours L4 L5 L6 L7 | L8 L9 L10 L11
sketch "Sketch11" plane through (0, 0, 0) normal (0, 1, 0) x (1, 0, 0)
  circle A0 centre (27, -54) radius 2.75
  circle A1 centre (27, -22) radius 2.75
  line L0 (17, -8) -> (17, -68)
  line L1 (37, -8) -> (37, -68)
  line L2 (17, -68) -> (37, -68)
  line L3 (0, -8) -> (93, -8)
  dimension "d180" = 5.5
  dimension "d181" = 5.5
  dimension "d182" = 32
  dimension "d183" = 10
  dimension "d184" = 10
  dimension "d185" = 10
  dimension "d186" = 14
  dimension "d187" = 14
  measures "d180" diameter of A0
  measures "d181" diameter of A1
  measures "d182" distance of A0.centre A1.centre
  measures "d183" distance of A1.centre L0
  measures "d184" distance of A0.centre L0
  measures "d185" distance of A0.centre L1
  measures "d186" distance of A0.centre L2
  measures "d187" distance of A1.centre L3
extrude "Extrude10" cut sketch "Sketch11" along normal blind 30 contours A0 | A1
sketch "Sketch12" plane through (0, 0, 0) normal (0, 1, 0) x (1, 0, 0)
  circle A0 centre (66, -54) radius 2.75
  circle A1 centre (66, -22) radius 2.75
  line L0 (93, -8) -> (0, -8)
  line L1 (76, -68) -> (56, -68)
  line L2 (76, -8) -> (76, -68)
  line L3 (56, -8) -> (56, -68)
  dimension "d190" = 5.5
  dimension "d191" = 5.5
  dimension "d193" = 32
  dimension "d194" = 14
  dimension "d195" = 14
  dimension "d196" = 10
  dimension "d197" = 10
  dimension "d198" = 10
  dimension "d199" = 10
  measures "d190" diameter of A0
  measures "d191" diameter of A1
  measures "d193" vertical distance of A0.centre A1.centre
  measures "d194" distance of A1.centre L0
  measures "d195" distance of A0.centre L1
  measures "d196" distance of A0.centre L2
  measures "d197" distance of A0.centre L3
  measures "d198" distance of A1.centre L2
  measures "d199" distance of A1.centre L3
extrude "Extrude11" cut sketch "Sketch12" along normal blind 600 from surface at 40 contours A0 | A1
sketch "Sketch13" plane through (0, 0, 0) normal (0, 1, 0) x (1, 0, 0)
  line L0 (44, -53) -> (86, -53)
  line L1 (86, -53) -> (86, -8)
  line L2 (86, -8) -> (44, -8)
  line L3 (44, -8) -> (44, -53)
  constraint horizontal L0
  constraint vertical L1
  constraint horizontal L2
  constraint vertical L3
extrude "Extrude12" cut sketch "Sketch13" along normal blind 25
sketch "Sketch14" plane through (0, 0, 8) normal (0, 0, 1) x (-1, 0, 0)
  circle A0 centre (-15, -30) radius 2.1
  circle A1 centre (-39, -30) radius 2.1
  circle A2 centre (-15, -48) radius 2.1
  circle A3 centre (-39, -48) radius 2.1
  circle A4 centre (-78, -48) radius 2.1
  circle A5 centre (-54, -30) radius 2.1
  circle A6 centre (-54, -48) radius 2.1
  circle A7 centre (-78, -30) radius 2.1
  line L0 (-17, -10) -> (-17, -20)
  line L1 (-17, -20) -> (-37, -20)
  line L2 (-37, -20) -> (-37, -10)
  line L3 (-37, -10) -> (-17, -10)
  line L4 (-56, -58) -> (-56, -68)
  line L5 (-56, -68) -> (-76, -68)
  line L6 (-76, -68) -> (-76, -58)
  line L7 (-76, -58) -> (-56, -58)
  line L8 (0, 0) -> (-93, 0)
  line L9 (-93, 0) -> (-93, -78)
  line L10 (-93, -78) -> (0, -78)
  line L11 (0, -78) -> (0, 0)
  line L12 (-52, -20) -> (-72, -20)
  line L13 (-72, -20) -> (-72, -10)
  line L14 (-72, -10) -> (-52, -10)
  line L15 (-52, -10) -> (-52, -20)
  line L16 (-52, -41.5) -> (-72, -41.5)
  line L17 (-72, -41.5) -> (-72, -36.5)
  line L18 (-72, -36.5) -> (-52, -36.5)
  line L19 (-52, -36.5) -> (-52, -41.5)
  dimension "d205" = 20
  dimension "d206" = 10
  dimension "d207" = 15
  dimension "d209" = 10
  dimension "d210" = 20
  dimension "d211" = 5
  dimension "d212" = 16.5
  dimension "d213" = 15
  dimension "d214" = 6.5
  dimension "d215" = 6.5
  constraint horizontal L12
  constraint vertical L13
  constraint horizontal L14
  constraint vertical L15
  constraint horizontal L16
  constraint vertical L17
  constraint horizontal L18
  constraint vertical L19
  measures "d205" distance of L12.start L12.end
  measures "d206" distance of L12 L14
  measures "d207" distance of L2 L15
  measures "d209" distance of L8 L14
  measures "d210" distance of L16.start L16.end
  measures "d211" distance of L16 L18
  measures "d212" distance of L12 L18
  measures "d213" distance of L2 L19
  measures "d214" distance of A5.centre L18
  measures "d215" distance of A6.centre L16
extrude "Extrude13" add sketch "Sketch14" along normal blind 45 contours L12 L13 L14 L15 | L16 L17 L18 L19
sketch "Sketch15" plane through (0, 0, 0) normal (0, 1, 0) x (1, 0, 0)
  circle A0 centre (62, -32) radius 2.75
  line L0 (0, -8) -> (93, -8)
  line L1 (52, -8) -> (52, -53)
  line L2 (72, -8) -> (72, -53)
  line L3 (52, -53) -> (72, -53)
  dimension "d218" = 5.5
  dimension "d219" = 24
  dimension "d220" = 10
  dimension "d221" = 10
  dimension "d222" = 21
  measures "d218" diameter of A0
  measures "d219" distance of A0.centre L0
  measures "d220" distance of A0.centre L1
  measures "d221" distance of A0.centre L2
  measures "d222" distance of A0.centre L3
extrude "Extrude14" cut sketch "Sketch15" along normal blind 45 contours A0
sketch "Sketch16" plane through (0, 0, 68) normal (0, 0, 1) x (-1, 0, 0)
  line L0 (-17, -10) -> (-37, -10)
  line L1 (-37, -10) -> (-37, -20)
  line L2 (-37, -20) -> (-17, -20)
  line L3 (-17, -20) -> (-17, -10)
extrude "Extrude15" cut sketch "Sketch16" against normal blind 60
extrude "Extrude16" cut 1 faces at (65.9315, 58, 64.2474) along direction (0, 1, 0) blind 20
sketch "sketch 5590" plane through (0, 0, 8) normal (0, 0, 1) x (-1, 0, 0)
  line L0 (-93, -78) -> (0, -78)
  line L1 (0, -78) -> (0, 0)
  line L2 (0, 0) -> (-93, 0)
  line L3 (-93, 0) -> (-93, -78)
  circle A0 centre (-78, -30) radius 2.1
  circle A1 centre (-54, -48) radius 2.1
  circle A2 centre (-54, -30) radius 2.1
  circle A3 centre (-78, -48) radius 2.1
  circle A4 centre (-39, -48) radius 2.1
  circle A5 centre (-15, -48) radius 2.1
  circle A6 centre (-39, -30) radius 2.1
  circle A7 centre (-15, -30) radius 2.1
  circle A8 centre (-41, -67) radius 2.75
  circle A9 centre (-41, -67) radius 2.75
extrude "Extrude17" cut sketch "sketch 5590" against normal blind 11 contours A8 A9
sketch "sketch 5742" plane through (0, 10, 0) normal (0, -1, 0) x (1, 0, 0)
  circle A0 centre (62, 32) radius 2.75
  line L0 (52, 8) -> (72, 8)
  line L1 (72, 8) -> (72, 53)
  line L2 (72, 53) -> (52, 53)
  line L3 (52, 53) -> (52, 8)
  line L4 (52, 53) -> (76, 53)
  line L5 (76, 53) -> (76, 8)
  line L6 (76, 8) -> (52, 8)
  line L7 (52, 8) -> (52, 53)
extrude "Extrude18" cut sketch "sketch 5742" against normal blind 35 contours L0 L1 L2 L3 L4 L6 L7
